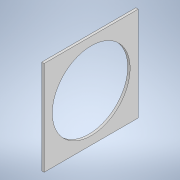
# Autodesk Inventor part: Mag_Shield_front
Saved by Autodesk Inventor 2022 (Build 260153000, 153)
## iProperties
Created: 2022-03-10
Part Number: Mag_Shield_front
Material: Generic
Document SubType Name: Modeling
Designer: Mlees
Density: 1 g/cm^3
Appearance: Default
Author: Mlees
Autodesk Inventor part; units mm, degrees
ref_plane "YZ Plane" through (0, 0, 0) normal (1, 0, 0) x (0, 1, 0)
ref_plane "XZ Plane" through (0, 0, 0) normal (0, 1, 0) x (-1, 0, 0)
ref_plane "XY Plane" through (0, 0, 0) normal (0, 0, 1) x (1, 0, 0)
sketch "Sketch1" plane through (0, 0, 0) normal (1, 0, 0) x (0, 1, 0)
  line L0 (0, 0) -> (38.75, 0)
  line L1 (38.75, 0) -> (38.75, -38.75)
  line L2 (38.75, -38.75) -> (0, -38.75)
  line L3 (0, -38.75) -> (0, 0)
  line L4 (0, -19.375) -> (19.375, -19.375)
  circle A0 centre (19.375, -19.375) radius 16
  dimension "d0" = 38.75
  dimension "d1" = 38.75
  dimension "d2" = 32
  constraints: 10 end point, 3 parallel, 1 centre point, 1 coincident, 1 horizontal, 1 midpoint, 1 perpendicular
  measures "d0" distance of L1.end L2.end
  measures "d1" distance of L0.end L1.end
  measures "d2" diameter of A0
extrude "Extrusion1" add sketch "Sketch1" along normal blind 1
body "Solid1"
